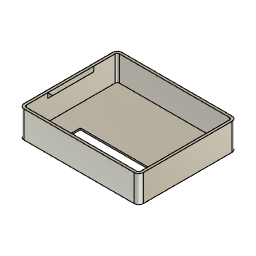
BoilerCase (Autodesk Fusion 360 design; units mm, degrees)
part number: Top
part number: Case
Autodesk Fusion 360 part; units mm, degrees
note: some values were not read from the file. Set by a fixed rule: which face or edge a step refers to.
sketch "Sketch1" plane through (0, 0, 0) normal (0, 0, 1) x (1, 0, 0) in component "Case"
  line L0 (0, 0) -> (77.7, 0)
  line L1 (77.7, 0) -> (77.7, -63.7)
  line L2 (77.7, -63.7) -> (0, -63.7)
  line L3 (0, -63.7) -> (0, 0)
  dimension "d7" = 77.7
  dimension "d8" = 63.7
  constraint horizontal L0
  constraint vertical L1
  constraint horizontal L2
  constraint vertical L3
  constraint coincident L0.start L3.end
  measures "d7" distance of L0.start L0.end
  measures "d8" distance of L0.start L2.end
extrude "Extrude1" add sketch "Sketch1" along normal blind 17.5 makes body 1 in component "Case"
fillet "Fillet1" radius 3 4 edges at (0, 0, 8.75) (77.7, 0, 8.75) (77.7, -63.7, 8.75) (0, -63.7, 8.75) on bodies 1 in component "Case"
shell "Shell1" thickness 1.6 removed faces 1 at (50.8, -42.4667, 17.5) on bodies 1 in component "Case"
sketch "Sketch2" plane through (76.1, 0, 0) normal (-1, 0, 0) x (0, -1, 0) in component "Case"
  line L0 (60.7, 1.6) -> (60.7, 17.5)
  line L1 (60.7, 17.5) -> (3, 17.5)
  line L2 (3, 17.5) -> (3, 1.6)
  line L3 (3, 1.6) -> (60.7, 1.6)
  line L4 (16.85, 17.5) -> (46.85, 17.5)
  line L5 (46.85, 17.5) -> (46.85, 14.3)
  line L6 (46.85, 14.3) -> (16.85, 14.3)
  line L7 (16.85, 14.3) -> (16.85, 17.5)
  line L8 (30, 19) -> (30.3564, 19) construction
  line L9 (31.85, 17.5) -> (31.85, 14.3) construction
  dimension "d15" = 3.2
  dimension "d16" = 30
  constraint horizontal L4
  constraint vertical L5
  constraint horizontal L6
  constraint vertical L7
  constraint coincident L1 L4.start
  constraint horizontal L8
  constraint midpoint L1 L9.start
  constraint midpoint L6 L9.end
  constraint vertical L9
  measures "d15" distance of L4 L6
  measures "d16" distance of L5 L7
extrude "Extrude2" add sketch "Sketch2" along normal blind 6 draft -45 contours L1 L4 L5 L6 L7 bodies 1 in component "Case"
ref_plane "WorkPlane1" through (38.85, -31.85, 8.75) normal (-1, 0, 0) x (0, -1, 0) in component "Case"
mirror "Mirror1" about plane through (38.85, -31.85, 8.75) normal (-1, 0, 0) of "Extrude2" in component "Case"
sketch "Sketch4" plane through (0, 0, 1.6) normal (0, 0, 1) x (-1, 0, 0) in component "Case"
  arc A0 (-1.6, 60.7) -> (-3, 62.1) centre (-3, 60.7) ccw
  line L0 (-3, 62.1) -> (-74.7, 62.1)
  arc A1 (-74.7, 62.1) -> (-76.1, 60.7) centre (-74.7, 60.7) ccw
  line L1 (-76.1, 60.7) -> (-76.1, 3)
  arc A2 (-76.1, 3) -> (-74.7, 1.6) centre (-74.7, 3) ccw
  line L2 (-74.7, 1.6) -> (-3, 1.6)
  arc A3 (-3, 1.6) -> (-1.6, 3) centre (-3, 3) ccw
  line L3 (-1.6, 3) -> (-1.6, 60.7)
  line L4 (-74.1, 39.6) -> (-15.6, 39.6)
  line L5 (-15.6, 39.6) -> (-15.6, 58.1)
  line L6 (-15.6, 58.1) -> (-74.1, 58.1)
  line L7 (-74.1, 58.1) -> (-74.1, 39.6)
  line L8 (-76.1, 60.7) -> (-76.1, 3)
  line L9 (-3, 62.1) -> (-74.7, 62.1)
  dimension "d29" = 58.5
  dimension "d30" = 18.5
  dimension "d31" = 2
  dimension "d32" = 4
  constraint horizontal L4
  constraint vertical L5
  constraint horizontal L6
  constraint vertical L7
  measures "d29" distance of L4.start L4.end
  measures "d30" distance of L4.start L6.end
  measures "d31" distance of L7 L8
  measures "d32" distance of L6 L9
extrude "Extrude3" cut sketch "Sketch4" against normal blind 4 contours L4 L5 L6 L7 bodies 1 in component "Case"
extrude "Extrude4" cut 1 faces at (31.1, -14.2667, 1.6) along direction (0, 0, -1) blind 0.6 on bodies 1 bodies 1 in component "Case"
sketch "Sketch1 (2)" plane through (0, 0, 17.5) normal (0, 0, 1) x (-1, 0, 0) in component "Top (1)"
  arc A0 (-1.6, 60.7) -> (-3, 62.1) centre (-3, 60.7) ccw
  line L0 (-1.6, 60.7) -> (-1.6, 46.85)
  line L1 (-1.6, 46.85) -> (-1.6, 16.85)
  line L2 (-1.6, 16.85) -> (-1.6, 3)
  arc A1 (-3, 1.6) -> (-1.6, 3) centre (-3, 3) ccw
  line L3 (-3, 1.6) -> (-74.7, 1.6)
  arc A2 (-76.1, 3) -> (-74.7, 1.6) centre (-74.7, 3) ccw
  line L4 (-76.1, 3) -> (-76.1, 16.85)
  line L5 (-76.1, 16.85) -> (-76.1, 46.85)
  line L6 (-76.1, 46.85) -> (-76.1, 60.7)
  arc A3 (-74.7, 62.1) -> (-76.1, 60.7) centre (-74.7, 60.7) ccw
  line L7 (-74.7, 62.1) -> (-3, 62.1)
  arc A4 (0, 60.7) -> (-3, 63.7) centre (-3, 60.7) ccw
  line L8 (-3, 63.7) -> (-74.7, 63.7)
  arc A5 (-74.7, 63.7) -> (-77.7, 60.7) centre (-74.7, 60.7) ccw
  line L9 (-77.7, 60.7) -> (-77.7, 3)
  arc A6 (-77.7, 3) -> (-74.7, 0) centre (-74.7, 3) ccw
  line L10 (-74.7, 0) -> (-3, 0)
  arc A7 (-3, 0) -> (0, 3) centre (-3, 3) ccw
  line L11 (0, 3) -> (0, 60.7)
extrude "Extrude1'" add sketch "Sketch1 (2)" along normal blind 2 separate body contours A0 L0 L1 L2 A1 L3 A2 L4 L5 L6 A3 L7 | A4 L8 A5 L9 A6 L10 A7 L11 makes body 2 in component "Top (1)"
sketch "Sketch2 (2)" plane through (0, 0, 17.5) normal (0, 0, -1) x (1, 0, 0) in component "Top (1)"
  line L0 (0, 60.7) -> (0, 3)
  arc A0 (0, 3) -> (3, 0) centre (3, 3) ccw
  line L1 (3, 0) -> (74.7, 0)
  arc A1 (74.7, 0) -> (77.7, 3) centre (74.7, 3) ccw
  line L2 (77.7, 3) -> (77.7, 60.7)
  arc A2 (77.7, 60.7) -> (74.7, 63.7) centre (74.7, 60.7) ccw
  line L3 (74.7, 63.7) -> (3, 63.7)
  arc A3 (3, 63.7) -> (0, 60.7) centre (3, 60.7) ccw
  line L4 (3, 2.1) -> (74.7, 2.1)
  arc A4 (74.7, 2.1) -> (75.6, 3) centre (74.7, 3) ccw
  line L5 (75.6, 3) -> (75.6, 60.7)
  arc A5 (75.6, 60.7) -> (74.7, 61.6) centre (74.7, 60.7) ccw
  line L6 (74.7, 61.6) -> (3, 61.6)
  arc A6 (3, 61.6) -> (2.1, 60.7) centre (3, 60.7) ccw
  line L7 (2.1, 60.7) -> (2.1, 3)
  arc A7 (2.1, 3) -> (3, 2.1) centre (3, 3) ccw
extrude "Extrude2'" add sketch "Sketch2 (2)" along normal blind 3.2 contours L4 A4 L5 A5 L6 A6 L7 A7 bodies 2 in component "Top (1)"
sketch "Sketch3" plane through (0, 0, 14.3) normal (0, 0, -1) x (1, 0, 0) in component "Top (1)"
  arc A0 (2.1, 3) -> (3, 2.1) centre (3, 3) ccw
  line L0 (3, 2.1) -> (74.7, 2.1)
  arc A1 (74.7, 2.1) -> (75.6, 3) centre (74.7, 3) ccw
  line L1 (75.6, 3) -> (75.6, 60.7)
  arc A2 (75.6, 60.7) -> (74.7, 61.6) centre (74.7, 60.7) ccw
  line L2 (74.7, 61.6) -> (3, 61.6)
  arc A3 (3, 61.6) -> (2.1, 60.7) centre (3, 60.7) ccw
  line L3 (2.1, 60.7) -> (2.1, 3)
  line L4 (73.6, 59.6) -> (4.1, 59.6)
  line L5 (4.1, 59.6) -> (4.1, 4.1)
  line L6 (4.1, 4.1) -> (73.6, 4.1)
  line L7 (73.6, 4.1) -> (73.6, 59.6)
  dimension "d42" = -2
extrude "Extrude3'" cut sketch "Sketch3" against normal blind 2 contours L4 L5 L6 L7 bodies 2 in component "Top (1)"
extrude "Extrude4'" cut sketch "Sketch2" along normal blind 2 draft -45 from surface at 0.5 contours L1 L4 L5 L6 L7 bodies 2 in component "Top (1)"
mirror "Mirror1'" about plane through (38.85, -31.85, 8.75) normal (-1, 0, 0) of "Extrude4'" in component "Top (1)"
sketch "Sketch4 (2)" plane through (0, 0, 19.5) normal (0, 0, 1) x (-1, 0, 0) in component "Top (1)"
  line L0 (0, 3) -> (0, 60.7)
  arc A0 (0, 60.7) -> (-3, 63.7) centre (-3, 60.7) ccw
  line L1 (-3, 63.7) -> (-74.7, 63.7)
  arc A1 (-74.7, 63.7) -> (-77.7, 60.7) centre (-74.7, 60.7) ccw
  line L2 (-77.7, 60.7) -> (-77.7, 3)
  arc A2 (-77.7, 3) -> (-74.7, 0) centre (-74.7, 3) ccw
  line L3 (-74.7, 0) -> (-3, 0)
  arc A3 (-3, 0) -> (0, 3) centre (-3, 3) ccw
  line L4 (-63.1, 7.6) -> (-66.6, 7.6)
  line L5 (-66.6, 7.6) -> (-66.6, 32.6)
  line L6 (-66.6, 32.6) -> (-63.1, 32.6)
  line L7 (-63.1, 32.6) -> (-63.1, 7.6)
  line L8 (-43.6, 7.6) -> (-40.1, 7.6)
  line L9 (-40.1, 7.6) -> (-40.1, 32.6)
  line L10 (-40.1, 32.6) -> (-43.6, 32.6)
  line L11 (-43.6, 32.6) -> (-43.6, 7.6)
  line L12 (-45.85, 12.6) -> (-60.85, 12.6)
  line L13 (-60.85, 12.6) -> (-60.85, 27.6)
  line L14 (-60.85, 27.6) -> (-45.85, 27.6)
  line L15 (-45.85, 27.6) -> (-45.85, 12.6)
  circle A4 centre (-61.1, 43.6) radius 3
  circle A5 centre (-26.6, 36.6) radius 3
  circle A6 centre (-26.6, 48.6) radius 3
  line L16 (-6.6, 22) -> (-15.6, 22)
  line L17 (-15.6, 22) -> (-15.6, 28)
  line L18 (-15.6, 28) -> (-6.6, 28)
  line L19 (-6.6, 28) -> (-6.6, 22)
  line L20 (-54.1, 49.1) -> (-65.1, 49.1)
  line L21 (-65.1, 49.1) -> (-65.1, 62.1)
  line L22 (-65.1, 62.1) -> (-54.1, 62.1)
  line L23 (-54.1, 62.1) -> (-54.1, 49.1)
  line L24 (-40.1, 49.1) -> (-51.1, 49.1)
  line L25 (-51.1, 49.1) -> (-51.1, 62.1)
  line L26 (-51.1, 62.1) -> (-40.1, 62.1)
  line L27 (-40.1, 62.1) -> (-40.1, 49.1)
  dimension "d50" = 6
  dimension "d51" = 6
  dimension "d52" = 6
  dimension "d53" = 25
  dimension "d54" = 3.5
  dimension "d55" = 15
  dimension "d56" = 15
  dimension "d57" = 3.5
  dimension "d58" = 25
  dimension "d59" = 7.6
  dimension "d60" = 7.6
  dimension "d61" = 19.5
  dimension "d62" = 11.1
  dimension "d63" = 2.25
  dimension "d64" = 2.25
  dimension "d65" = 5
  dimension "d66" = 5
  dimension "d67" = 16.6
  dimension "d68" = 20.1
  dimension "d69" = 15.1
  dimension "d70" = 12
  dimension "d71" = 26.6
  dimension "d72" = 26.6
  dimension "d73" = 22
  dimension "d74" = 6.6
  dimension "d75" = 9
  dimension "d76" = 6
  dimension "d85" = 11
  dimension "d86" = 13
  dimension "d87" = 1.6
  dimension "d88" = 11
  dimension "d89" = 13
  dimension "d90" = 1.6
  dimension "d91" = 3
  dimension "d92" = 12.6
  constraint horizontal L4
  constraint vertical L5
  constraint horizontal L6
  constraint vertical L7
  constraint horizontal L8
  constraint vertical L9
  constraint horizontal L10
  constraint vertical L11
  constraint horizontal L12
  constraint vertical L13
  constraint horizontal L14
  constraint vertical L15
  constraint horizontal L16
  constraint vertical L17
  constraint horizontal L18
  constraint vertical L19
  constraint horizontal L20
  constraint vertical L21
  constraint horizontal L22
  constraint vertical L23
  constraint horizontal L24
  constraint vertical L25
  constraint horizontal L26
  constraint vertical L27
  measures "d50" diameter of A5
  measures "d51" diameter of A6
  measures "d52" diameter of A4
  measures "d53" distance of L8 L10
  measures "d54" distance of L9 L11
  measures "d55" distance of L12 L14
  measures "d56" distance of L13 L15
  measures "d57" distance of L5 L7
  measures "d58" distance of L4 L6
  measures "d59" distance of L3 L4
  measures "d60" distance of L3 L8
  measures "d61" distance of L7 L11
  measures "d62" distance of L2 L5
  measures "d63" distance of L7 L13
  measures "d64" distance of L11 L15
  measures "d65" distance of L4 L12
  measures "d66" distance of L6 L14
  measures "d67" distance of L2 A4.centre
  measures "d68" distance of L1 A4.centre
  measures "d69" distance of L1 A6.centre
  measures "d70" vertical distance of A5.centre A6.centre
  measures "d71" distance of L0 A6.centre
  measures "d72" distance of L0 A5.centre
  measures "d73" distance of L3 L16.start
  measures "d74" distance of L0 L19
  measures "d75" distance of L17 L19
  measures "d76" distance of L16 L18
  measures "d85" distance of L20.start L20.end
  measures "d86" distance of L20.start L22.end
  measures "d87" distance of L1 L22
  measures "d88" distance of L24.start L24.end
  measures "d89" distance of L24.start L26.end
  measures "d90" distance of L1 L26
  measures "d91" distance of L23 L25
  measures "d92" distance of L2 L21
extrude "Extrude5" cut sketch "Sketch4 (2)" against normal blind 9 contours L4 L5 L6 L7 | L8 L9 L10 L11 | L12 L13 L14 L15 | A4 | A5 | A6 bodies 2 in component "Top (1)"
extrude "Extrude6" cut 1 faces at (23.3775, -15.1251, 16.3) along direction (0, 0, 1) blind 1.5 on bodies 2 bodies 2 in component "Top (1)"
extrude "Extrude7" cut sketch "Sketch4 (2)" against normal blind 1.2 contours L16 L17 L18 L19 bodies 2 in component "Top (1)"
extrude "Extrude8" cut 1 faces at (9.6, -26, 18.3) along direction (0, 0, -1) blind 0.15 on bodies 2 bodies 2 in component "Top (1)"
extrude "Extrude9" cut sketch "Sketch4 (2)" against normal blind 6 contours L20 L21 L22 L23 | L24 L25 L26 L27 bodies 2 in component "Top (1)"
sketch "Sketch5" plane through (0, 0, 14.3) normal (0, 0, -1) x (1, 0, 0) in component "Top (1)"
  line L0 (65.1, 61.6) -> (65.1, 59.6)
  line L1 (65.1, 59.6) -> (73.6, 59.6)
  line L2 (73.6, 59.6) -> (73.6, 4.1)
  line L3 (73.6, 4.1) -> (4.1, 4.1)
  line L4 (4.1, 4.1) -> (4.1, 59.6)
  line L5 (4.1, 59.6) -> (40.1, 59.6)
  line L6 (40.1, 59.6) -> (40.1, 61.6)
  line L7 (40.1, 61.6) -> (3, 61.6)
  arc A0 (3, 61.6) -> (2.1, 60.7) centre (3, 60.7) ccw
  line L8 (2.1, 60.7) -> (2.1, 46.85)
  line L9 (2.1, 46.85) -> (2.1, 16.85)
  line L10 (2.1, 16.85) -> (2.1, 3)
  arc A1 (2.1, 3) -> (3, 2.1) centre (3, 3) ccw
  line L11 (3, 2.1) -> (74.7, 2.1)
  arc A2 (74.7, 2.1) -> (75.6, 3) centre (74.7, 3) ccw
  line L12 (75.6, 3) -> (75.6, 16.85)
  line L13 (75.6, 16.85) -> (75.6, 46.85)
  line L14 (75.6, 46.85) -> (75.6, 60.7)
  arc A3 (75.6, 60.7) -> (74.7, 61.6) centre (74.7, 60.7) ccw
  line L15 (74.7, 61.6) -> (65.1, 61.6)
  line L16 (4.1, 10.1) -> (3, 10.1)
  line L17 (3, 10.1) -> (3, 17.3539)
  line L18 (3, 17.3539) -> (4.1, 17.3539)
  line L19 (4.1, 17.3539) -> (4.1, 10.1)
  dimension "d95" = 8
  constraint horizontal L16
  constraint vertical L17
  constraint horizontal L18
  constraint vertical L19
  constraint coincident L4 L16.start
  measures "d95" distance of L11 L16
extrude "Extrude10" cut sketch "Sketch5" against normal blind 2 contours L4 L16 L17 L18 L19 bodies 2 in component "Top (1)"
ref_plane "WorkPlane1" through (38.85, -31.85, 8.75) normal (0, -1, 0) x (1, 0, 0)
sketch "Sketch6" plane through (0, 0, 17.8) normal (0, 0, -1) x (1, 0, 0) in component "Top (1)"
  line L0 (65.1, 59.6) -> (65.1, 49.1)
  line L1 (65.1, 49.1) -> (54.1, 49.1)
  line L2 (54.1, 49.1) -> (54.1, 59.6)
  line L3 (54.1, 59.6) -> (51.1, 59.6)
  line L4 (51.1, 59.6) -> (51.1, 49.1)
  line L5 (51.1, 49.1) -> (40.1, 49.1)
  line L6 (40.1, 49.1) -> (40.1, 59.6)
  line L7 (40.1, 59.6) -> (4.1, 59.6)
  line L8 (4.1, 59.6) -> (4.1, 4.1)
  line L9 (4.1, 4.1) -> (73.6, 4.1)
  line L10 (73.6, 4.1) -> (73.6, 59.6)
  line L11 (73.6, 59.6) -> (65.1, 59.6)
  circle A0 centre (26.6, 36.6) radius 3
  line L12 (60.85, 27.6) -> (60.85, 12.6)
  line L13 (60.85, 12.6) -> (45.85, 12.6)
  line L14 (45.85, 12.6) -> (45.85, 27.6)
  line L15 (45.85, 27.6) -> (60.85, 27.6)
  line L16 (66.6, 32.6) -> (66.6, 7.6)
  line L17 (66.6, 7.6) -> (63.1, 7.6)
  line L18 (63.1, 7.6) -> (63.1, 32.6)
  line L19 (63.1, 32.6) -> (66.6, 32.6)
  circle A1 centre (26.6, 48.6) radius 3
  line L20 (43.6, 7.6) -> (40.1, 7.6)
  line L21 (40.1, 7.6) -> (40.1, 32.6)
  line L22 (40.1, 32.6) -> (43.6, 32.6)
  line L23 (43.6, 32.6) -> (43.6, 7.6)
  circle A2 centre (61.1, 43.6) radius 3
  line L24 (20.5409, 59.6) -> (4.1, 59.6)
  line L25 (4.1, 59.6) -> (4.1, 31.2604)
  line L26 (4.1, 31.2604) -> (20.5409, 31.2604)
  line L27 (20.5409, 31.2604) -> (20.5409, 59.6)
  constraint horizontal L24
  constraint vertical L25
  constraint horizontal L26
  constraint vertical L27
  constraint coincident L8 L25.end
  constraint coincident L7 L24.start
extrude "Extrude11" cut sketch "Sketch6" against normal blind 1 contours L7 L8 L24 L25 L26 L27 bodies 2 in component "Top (1)"
extrude "Extrude12" cut 1 faces at (9.6, -26, 18.15) along direction (0, 0, -1) blind 0.2 on bodies 2 bodies 2 in component "Top (1)"
component "Enclosure" placed x (1, 0, 0) y (0, 1, 0) z (0, 0, 1) at (0, 0, 0)
component "Top (1)" placed x (1, 0, 0) y (0, 1, 0) z (0, 0, 1) at (0, 0, 0) in component "Enclosure"
component "Case" placed x (1, 0, 0) y (0, 1, 0) z (0, 0, 1) at (0, 0, 0) in component "Enclosure"
equation "Width = 60 mm"
equation "Length = 74 mm"
equation "Height = 17 mm"
equation "Shell = 1.6 mm"
equation "gap = 0.5 mm"
equation "d7 = Length + 2 * Shell + gap"
equation "d8 = Width + 2 * Shell + gap"
equation "d9 = Height + gap"
equation "Fillet = 3 mm"
equation "d13 = Fillet"
equation "d14 = Shell"
equation "d15 = 2 * Shell"
equation "d16 = Width / 2"
equation "BatteryWidth = 58 mm"
equation "BatteryLength = 18 mm"
equation "BatteryOffsetH = 2 mm"
equation "BatteryOffsetV = 4 mm"
equation "d29 = BatteryWidth + gap"
equation "d30 = BatteryLength + gap"
equation "d31 = BatteryOffsetH"
equation "d32 = BatteryOffsetV"
equation "d39 = -( Shell + gap )"
equation "d40 = 2 * Shell"
equation "d59 = 6 mm + Shell"
equation "d60 = 6 mm + Shell"
equation "d62 = 9.5 mm + Shell"
equation "d67 = 15 mm + Shell"
equation "d68 = 18.5 mm + Shell"
equation "d69 = 13.5 mm + Shell"
equation "d71 = 25 mm + Shell"
equation "d72 = 25 mm + Shell"
equation "d74 = 5 mm + Shell"
equation "d87 = Shell"
equation "d90 = Shell"
equation "d92 = 11 mm + Shell"
